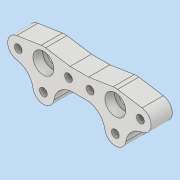
# Autodesk Inventor part: carriageIdlerPinionExtension
Saved by Autodesk Inventor 2017 (Build 210142000, 142)
## iProperties
Created: 2016-12-14
Part Number: carriageIdlerPinionExtension
Material: ABS Plastic
Document SubType Name: Modeling
Designer: techn
Density: 1.06 g/cm^3
Appearance: Smooth - White
Author: techn
Autodesk Inventor part; units mm, degrees
ref_plane "YZ Plane" through (0, 0, 0) normal (1, 0, 0) x (0, 1, 0)
ref_plane "XZ Plane" through (0, 0, 0) normal (0, 1, 0) x (-1, 0, 0)
ref_plane "XY Plane" through (0, 0, 0) normal (0, 0, 1) x (1, 0, 0)
sketch "Sketch5" plane through (0, 0, 0) normal (0, 0, 1) x (1, 0, 0)
  line L0 (0, 0) -> (8.255, 0)
  circle A0 centre (8.255, 0) radius 1.27
  circle A1 centre (0, -8.255) radius 1.27
  circle A2 centre (-8.255, 0) radius 1.27
  line L1 (0, 0) -> (-23.6329, 0)
  line L2 (-23.6329, 0) -> (-15.3779, 0)
  circle A3 centre (-15.3779, 0) radius 1.27
  circle A4 centre (-23.6329, -8.255) radius 1.27
  circle A5 centre (-31.8879, 0) radius 1.27
  circle A6 centre (-31.8879, 0) radius 3.4925
  circle A7 centre (-23.6329, -8.255) radius 3.4925
  circle A8 centre (-15.3779, 0) radius 3.4925
  circle A9 centre (-8.255, 0) radius 3.4925
  circle A10 centre (0, -8.255) radius 3.4925
  circle A11 centre (8.255, 0) radius 3.4925
  circle A12 centre (-23.6329, 0) radius 4.7625
  circle A13 centre (0, 0) radius 4.7625
  line L3 (-32.4252, 3.4509) -> (-24.3656, 4.7058)
  line L4 (-22.9002, 4.7058) -> (-14.8406, 3.4509)
  line L5 (-8.7923, 3.4509) -> (-0.7327, 4.7058)
  line L6 (0.7327, 4.7058) -> (8.7923, 3.4509)
  arc A14 (8.7788, -3.453) -> (3.453, -8.7788) centre (9.7312, -9.7312) ccw
  arc A15 (-3.453, -8.7788) -> (-8.7788, -3.453) centre (-9.7312, -9.7312) ccw
  arc A16 (-14.8541, -3.453) -> (-20.1799, -8.7788) centre (-13.9017, -9.7312) ccw
  arc A17 (-27.0859, -8.7788) -> (-32.4117, -3.453) centre (-33.3641, -9.7312) ccw
  line L7 (-14.8406, 3.4509) -> (-8.7923, 3.4509)
  line L8 (-14.8541, -3.453) -> (-8.7788, -3.453)
  dimension "d45" = 8.255
  dimension "d46" = 2.54
  dimension "d49" = 180
  dimension "d51" = 23.6329
  dimension "d52" = 8.255
  dimension "d53" = 2.54
  dimension "d56" = 180
  dimension "d58" = 6.985
  dimension "d59" = 6.985
  dimension "d60" = 6.985
  dimension "d61" = 6.985
  dimension "d62" = 6.985
  dimension "d63" = 6.985
  dimension "d64" = 9.525
  dimension "d65" = 9.525
  dimension "d66" = 6.35
  dimension "d67" = 6.35
  dimension "d68" = 6.35
  dimension "d69" = 6.35
  constraints: 25 point on circle, 18 centre point, 18 end point, 16 tangent, 10 coincident, 3 horizontal, 1 point on line, 10 other
  measures "d45" distance of L0.start L0.end
  measures "d46" diameter of A0
  measures "d51" distance of L0.start L1.end
  measures "d52" distance of L1.end L2.end
  measures "d53" diameter of A3
  measures "d58" diameter of A6
  measures "d59" diameter of A7
  measures "d60" diameter of A8
  measures "d61" diameter of A9
  measures "d62" diameter of A10
  measures "d63" diameter of A11
  measures "d64" diameter of A12
  measures "d65" diameter of A13
  measures "d66" radius of A17
  measures "d67" radius of A16
  measures "d68" radius of A15
  measures "d69" radius of A14
extrude "Extrusion7" add sketch "Sketch5" along normal blind 6.985 contours L1 A13 L0 | L0 A13 L1 | A13 L6 A11 | A11 | A11 A14 A10 A13 | A9 L1 A2 | L1 A2 A9 | A13 A10 A15 A9 | A9 L5 A13 | A10 | A9 L1 A8 L7 | L8 A8 L1 A9 | A8 L1 A3 | A8 A12 L4 | A16 A7 A12 A8 | A8 L1 A3 | A12 | A7 | A7 A17 A6 A12 | A12 A6 L3 | A6
sketch "Sketch6" plane through (0, 0, 6.985) normal (0, 0, 1) x (1, 0, 0)
  circle A0 centre (0, 0) radius 1.8415
  circle A1 centre (0, 0) radius 3.429
  circle A2 centre (-23.6329, 0) radius 1.8415
  circle A3 centre (-23.6329, 0) radius 3.429
  dimension "d72" = 3.683
  dimension "d73" = 6.858
  dimension "d74" = 23.6329
  dimension "d75" = 3.683
  dimension "d76" = 6.858
  constraints: 4 centre point, 4 coincident
  measures "d72" diameter of A0
  measures "d73" diameter of A1
  measures "d74" distance of point (0, 0) point (-23.633, 0)
  measures "d75" diameter of A2
  measures "d76" diameter of A3
extrude "Extrusion8" cut sketch "Sketch6" against normal through all contours A0 | A2
extrude "Extrusion9" cut sketch "Sketch6" against normal blind 3.175
equation "\"d59\" = d58"
equation "\"d60\" = d58"
equation "\"d61\" = d58"
equation "\"d62\" = d58"
equation "\"d63\" = d58"
equation "\"d67\" = d66"
equation "\"d68\" = d66"
equation "\"d69\" = d66"
body "Solid3"
